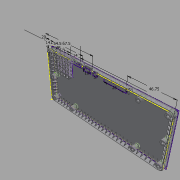
# Autodesk Inventor part: base
Saved by Autodesk Inventor 2019 (Build 230136000, 136)
## iProperties
Created: 2019-09-09
Part Number: base
Material: Generic
Document SubType Name: Modeling
Designer: jon
Density: 1 g/cm^3
Appearance: Default
Author: jon
Autodesk Inventor part; units mm, degrees
ref_plane "YZ Plane" through (0, 0, 0) normal (1, 0, 0) x (0, 1, 0)
ref_plane "XZ Plane" through (0, 0, 0) normal (0, 1, 0) x (-1, 0, 0)
ref_plane "XY Plane" through (0, 0, 0) normal (0, 0, 1) x (1, 0, 0)
sketch "Sketch1" plane through (0, 0, 0) normal (0, 0, 1) x (1, 0, 0)
  line L0 (0, 0) -> (154, 0)
  line L1 (154, 0) -> (154, 68)
  line L2 (154, 68) -> (0, 68)
  line L3 (0, 68) -> (0, 0)
  line L4 (1, 67) -> (153, 67)
  line L5 (153, 67) -> (153, 1)
  line L6 (153, 1) -> (1, 1)
  line L7 (1, 1) -> (1, 67)
  line L8 (1, 67) -> (8, 67)
  line L9 (1, 60) -> (1, 67)
  line L10 (1, 1) -> (8, 1)
  line L11 (1, 8) -> (1, 1)
  line L12 (153, 1) -> (146, 1)
  line L13 (153, 8) -> (153, 1)
  line L14 (153, 67) -> (146, 67)
  line L15 (153, 60) -> (153, 67)
  line L16 (30.5, 1) -> (37.5, 1)
  line L17 (116.5, 1) -> (123.5, 1)
  line L18 (116.5, 67) -> (123.5, 67)
  line L19 (30.5, 67) -> (37.5, 67)
  line L20 (1, 30.5) -> (1, 37.5)
  line L21 (153, 30.5) -> (153, 37.5)
  dimension "d0" = 154
  dimension "d1" = 68
  dimension "d2" = 1
  dimension "d3" = 1
  dimension "d4" = 1
  dimension "d123" = 1
  constraints: 44 end point, 10 horizontal, 6 point on line, 4 parallel, 2 perpendicular
  measures "d0" distance of L2.end L1.end
  measures "d1" distance of L1.end L0.end
  measures "d2" distance between parallel lines of L3 L7
  measures "d3" distance between parallel lines of L2 L4
  measures "d4" distance between parallel lines of L0 L6
  measures "d123" distance between parallel lines of L1 L5
extrude "Extrusion1" add sketch "Sketch1" along normal blind 6.4
extrude "Extrusion2" add sketch "Sketch1" against normal blind 1.3 contours L3 L2 L1 L0 | L4 L5 L6 L7
sketch "Sketch2" plane through (0, 0, 6.4) normal (0, 0, 1) x (1, 0, 0)
  line L0 (0, 68) -> (0, 0) projected
  line L1 (0, 0) -> (154, 0) projected
  line L2 (0, 68) -> (154, 68)
  line L3 (154, 68) -> (154, 0)
  line L4 (154, 0) -> (0, 0)
  line L5 (0, 0) -> (0, 68)
  line L6 (153.65, 67.65) -> (0.35, 67.65)
  line L7 (0.35, 67.65) -> (0.35, 0.35)
  line L8 (0.35, 0.35) -> (153.65, 0.35)
  line L9 (153.65, 0.35) -> (153.65, 67.65)
  dimension "d42" = 0.35
  constraints: 16 end point, 4 parallel, 2 perpendicular, 1 horizontal, 3 other
  measures "d42" distance between parallel lines of L2 L6
extrude "Extrusion3" cut sketch "Sketch2" against normal blind 1
fillet "Fillet2" radius 0.5 4 edges at (153, 34, 0) (77, 67, 0) (1, 34, 0) (77, 1, 0)
fillet "Fillet3" radius 4 8 edges at (152.8536, 1.1464, 0.1464) (153, 1, 3.45) (152.8536, 66.8536, 0.1464) (153, 67, 3.45) (1.1464, 1.1464, 0.1464) (1, 1, 3.45) (1.1464, 66.8536, 0.1464) (1, 67, 3.45)
fillet "Fillet9" radius 4.65 4 edges at (153.65, 0.35, 5.9) (153.65, 67.65, 5.9) (0.35, 67.65, 5.9) (0.35, 0.35, 5.9)
fillet "Fillet4" radius 5 4 edges at (154, 68, 2.05) (154, 0, 2.05) (0, 0, 2.05) (0, 68, 2.05)
sketch "Sketch10" plane through (0, 0, 0) normal (0, 0, 1) x (1, 0, 0)
  line L0 (149, 67) -> (5, 67) projected
  line L1 (5.25, 67) -> (4.75, 67)
  line L2 (4.75, 67) -> (4.75, 62)
  line L3 (4.75, 62) -> (5.25, 62)
  line L4 (5.25, 62) -> (5.25, 67)
  line L5 (0, 5) -> (0, 63) projected
  line L6 (5, 1) -> (149, 1) projected
  line L7 (5.25, 1) -> (4.75, 1)
  line L8 (4.75, 1) -> (4.75, 6)
  line L9 (4.75, 6) -> (5.25, 6)
  line L10 (5.25, 6) -> (5.25, 1)
  line L11 (10.215, 67) -> (9.715, 67)
  line L12 (9.715, 67) -> (9.715, 62)
  line L13 (9.715, 62) -> (10.215, 62)
  line L14 (10.215, 62) -> (10.215, 67)
  line L15 (10.215, 1) -> (9.715, 1)
  line L16 (9.715, 1) -> (9.715, 6)
  line L17 (9.715, 6) -> (10.215, 6)
  line L18 (10.215, 6) -> (10.215, 1)
  line L19 (15.18, 67) -> (14.68, 67)
  line L20 (14.68, 67) -> (14.68, 62)
  line L21 (14.68, 62) -> (15.18, 62)
  line L22 (15.18, 62) -> (15.18, 67)
  line L23 (15.18, 1) -> (14.68, 1)
  line L24 (14.68, 1) -> (14.68, 6)
  line L25 (14.68, 6) -> (15.18, 6)
  line L26 (15.18, 6) -> (15.18, 1)
  line L27 (20.145, 67) -> (19.645, 67)
  line L28 (19.645, 67) -> (19.645, 62)
  line L29 (19.645, 62) -> (20.145, 62)
  line L30 (20.145, 62) -> (20.145, 67)
  line L31 (20.145, 1) -> (19.645, 1)
  line L32 (19.645, 1) -> (19.645, 6)
  line L33 (19.645, 6) -> (20.145, 6)
  line L34 (20.145, 6) -> (20.145, 1)
  line L35 (25.11, 67) -> (24.61, 67)
  line L36 (24.61, 67) -> (24.61, 62)
  line L37 (24.61, 62) -> (25.11, 62)
  line L38 (25.11, 62) -> (25.11, 67)
  line L39 (25.11, 1) -> (24.61, 1)
  line L40 (24.61, 1) -> (24.61, 6)
  line L41 (24.61, 6) -> (25.11, 6)
  line L42 (25.11, 6) -> (25.11, 1)
  line L43 (30.075, 67) -> (29.575, 67)
  line L44 (29.575, 67) -> (29.575, 62)
  line L45 (29.575, 62) -> (30.075, 62)
  line L46 (30.075, 62) -> (30.075, 67)
  line L47 (30.075, 1) -> (29.575, 1)
  line L48 (29.575, 1) -> (29.575, 6)
  line L49 (29.575, 6) -> (30.075, 6)
  line L50 (30.075, 6) -> (30.075, 1)
  line L51 (35.04, 67) -> (34.54, 67)
  line L52 (34.54, 67) -> (34.54, 62)
  line L53 (34.54, 62) -> (35.04, 62)
  line L54 (35.04, 62) -> (35.04, 67)
  line L55 (35.04, 1) -> (34.54, 1)
  line L56 (34.54, 1) -> (34.54, 6)
  line L57 (34.54, 6) -> (35.04, 6)
  line L58 (35.04, 6) -> (35.04, 1)
  line L59 (40.005, 67) -> (39.505, 67)
  line L60 (39.505, 67) -> (39.505, 62)
  line L61 (39.505, 62) -> (40.005, 62)
  line L62 (40.005, 62) -> (40.005, 67)
  line L63 (40.005, 1) -> (39.505, 1)
  line L64 (39.505, 1) -> (39.505, 6)
  line L65 (39.505, 6) -> (40.005, 6)
  line L66 (40.005, 6) -> (40.005, 1)
  line L67 (44.97, 67) -> (44.47, 67)
  line L68 (44.47, 67) -> (44.47, 62)
  line L69 (44.47, 62) -> (44.97, 62)
  line L70 (44.97, 62) -> (44.97, 67)
  line L71 (44.97, 1) -> (44.47, 1)
  line L72 (44.47, 1) -> (44.47, 6)
  line L73 (44.47, 6) -> (44.97, 6)
  line L74 (44.97, 6) -> (44.97, 1)
  line L75 (49.935, 67) -> (49.435, 67)
  line L76 (49.435, 67) -> (49.435, 62)
  line L77 (49.435, 62) -> (49.935, 62)
  line L78 (49.935, 62) -> (49.935, 67)
  line L79 (49.935, 1) -> (49.435, 1)
  line L80 (49.435, 1) -> (49.435, 6)
  line L81 (49.435, 6) -> (49.935, 6)
  line L82 (49.935, 6) -> (49.935, 1)
  line L83 (54.9, 67) -> (54.4, 67)
  line L84 (54.4, 67) -> (54.4, 62)
  line L85 (54.4, 62) -> (54.9, 62)
  line L86 (54.9, 62) -> (54.9, 67)
  line L87 (54.9, 1) -> (54.4, 1)
  line L88 (54.4, 1) -> (54.4, 6)
  line L89 (54.4, 6) -> (54.9, 6)
  line L90 (54.9, 6) -> (54.9, 1)
  line L91 (59.865, 67) -> (59.365, 67)
  line L92 (59.365, 67) -> (59.365, 62)
  line L93 (59.365, 62) -> (59.865, 62)
  line L94 (59.865, 62) -> (59.865, 67)
  line L95 (59.865, 1) -> (59.365, 1)
  line L96 (59.365, 1) -> (59.365, 6)
  line L97 (59.365, 6) -> (59.865, 6)
  line L98 (59.865, 6) -> (59.865, 1)
  line L99 (64.83, 67) -> (64.33, 67)
  line L100 (64.33, 67) -> (64.33, 62)
  line L101 (64.33, 62) -> (64.83, 62)
  line L102 (64.83, 62) -> (64.83, 67)
  line L103 (64.83, 1) -> (64.33, 1)
  line L104 (64.33, 1) -> (64.33, 6)
  line L105 (64.33, 6) -> (64.83, 6)
  line L106 (64.83, 6) -> (64.83, 1)
  line L107 (69.795, 67) -> (69.295, 67)
  line L108 (69.295, 67) -> (69.295, 62)
  line L109 (69.295, 62) -> (69.795, 62)
  line L110 (69.795, 62) -> (69.795, 67)
  line L111 (69.795, 1) -> (69.295, 1)
  line L112 (69.295, 1) -> (69.295, 6)
  line L113 (69.295, 6) -> (69.795, 6)
  line L114 (69.795, 6) -> (69.795, 1)
  line L115 (74.76, 67) -> (74.26, 67)
  line L116 (74.26, 67) -> (74.26, 62)
  line L117 (74.26, 62) -> (74.76, 62)
  line L118 (74.76, 62) -> (74.76, 67)
  line L119 (74.76, 1) -> (74.26, 1)
  line L120 (74.26, 1) -> (74.26, 6)
  line L121 (74.26, 6) -> (74.76, 6)
  line L122 (74.76, 6) -> (74.76, 1)
  line L123 (79.725, 67) -> (79.225, 67)
  line L124 (79.225, 67) -> (79.225, 62)
  line L125 (79.225, 62) -> (79.725, 62)
  line L126 (79.725, 62) -> (79.725, 67)
  line L127 (79.725, 1) -> (79.225, 1)
  line L128 (79.225, 1) -> (79.225, 6)
  line L129 (79.225, 6) -> (79.725, 6)
  line L130 (79.725, 6) -> (79.725, 1)
  line L131 (84.69, 67) -> (84.19, 67)
  line L132 (84.19, 67) -> (84.19, 62)
  line L133 (84.19, 62) -> (84.69, 62)
  line L134 (84.69, 62) -> (84.69, 67)
  line L135 (84.69, 1) -> (84.19, 1)
  line L136 (84.19, 1) -> (84.19, 6)
  line L137 (84.19, 6) -> (84.69, 6)
  line L138 (84.69, 6) -> (84.69, 1)
  line L139 (89.655, 67) -> (89.155, 67)
  line L140 (89.155, 67) -> (89.155, 62)
  line L141 (89.155, 62) -> (89.655, 62)
  line L142 (89.655, 62) -> (89.655, 67)
  line L143 (89.655, 1) -> (89.155, 1)
  line L144 (89.155, 1) -> (89.155, 6)
  line L145 (89.155, 6) -> (89.655, 6)
  line L146 (89.655, 6) -> (89.655, 1)
  line L147 (94.62, 67) -> (94.12, 67)
  line L148 (94.12, 67) -> (94.12, 62)
  line L149 (94.12, 62) -> (94.62, 62)
  line L150 (94.62, 62) -> (94.62, 67)
  line L151 (94.62, 1) -> (94.12, 1)
  line L152 (94.12, 1) -> (94.12, 6)
  line L153 (94.12, 6) -> (94.62, 6)
  line L154 (94.62, 6) -> (94.62, 1)
  line L155 (99.585, 67) -> (99.085, 67)
  line L156 (99.085, 67) -> (99.085, 62)
  line L157 (99.085, 62) -> (99.585, 62)
  line L158 (99.585, 62) -> (99.585, 67)
  line L159 (99.585, 1) -> (99.085, 1)
  line L160 (99.085, 1) -> (99.085, 6)
  line L161 (99.085, 6) -> (99.585, 6)
  line L162 (99.585, 6) -> (99.585, 1)
  line L163 (104.55, 67) -> (104.05, 67)
  line L164 (104.05, 67) -> (104.05, 62)
  line L165 (104.05, 62) -> (104.55, 62)
  line L166 (104.55, 62) -> (104.55, 67)
  line L167 (104.55, 1) -> (104.05, 1)
  line L168 (104.05, 1) -> (104.05, 6)
  line L169 (104.05, 6) -> (104.55, 6)
  line L170 (104.55, 6) -> (104.55, 1)
  line L171 (109.515, 67) -> (109.015, 67)
  line L172 (109.015, 67) -> (109.015, 62)
  line L173 (109.015, 62) -> (109.515, 62)
  line L174 (109.515, 62) -> (109.515, 67)
  line L175 (109.515, 1) -> (109.015, 1)
  line L176 (109.015, 1) -> (109.015, 6)
  line L177 (109.015, 6) -> (109.515, 6)
  line L178 (109.515, 6) -> (109.515, 1)
  line L179 (114.48, 67) -> (113.98, 67)
  line L180 (113.98, 67) -> (113.98, 62)
  line L181 (113.98, 62) -> (114.48, 62)
  line L182 (114.48, 62) -> (114.48, 67)
  line L183 (114.48, 1) -> (113.98, 1)
  line L184 (113.98, 1) -> (113.98, 6)
  line L185 (113.98, 6) -> (114.48, 6)
  line L186 (114.48, 6) -> (114.48, 1)
  line L187 (119.445, 67) -> (118.945, 67)
  line L188 (118.945, 67) -> (118.945, 62)
  line L189 (118.945, 62) -> (119.445, 62)
  line L190 (119.445, 62) -> (119.445, 67)
  line L191 (119.445, 1) -> (118.945, 1)
  line L192 (118.945, 1) -> (118.945, 6)
  line L193 (118.945, 6) -> (119.445, 6)
  line L194 (119.445, 6) -> (119.445, 1)
  line L195 (124.41, 67) -> (123.91, 67)
  line L196 (123.91, 67) -> (123.91, 62)
  line L197 (123.91, 62) -> (124.41, 62)
  line L198 (124.41, 62) -> (124.41, 67)
  line L199 (124.41, 1) -> (123.91, 1)
  line L200 (123.91, 1) -> (123.91, 6)
  line L201 (123.91, 6) -> (124.41, 6)
  line L202 (124.41, 6) -> (124.41, 1)
  line L203 (129.375, 67) -> (128.875, 67)
  line L204 (128.875, 67) -> (128.875, 62)
  line L205 (128.875, 62) -> (129.375, 62)
  line L206 (129.375, 62) -> (129.375, 67)
  line L207 (129.375, 1) -> (128.875, 1)
  line L208 (128.875, 1) -> (128.875, 6)
  line L209 (128.875, 6) -> (129.375, 6)
  line L210 (129.375, 6) -> (129.375, 1)
  line L211 (134.34, 67) -> (133.84, 67)
  line L212 (133.84, 67) -> (133.84, 62)
  line L213 (133.84, 62) -> (134.34, 62)
  line L214 (134.34, 62) -> (134.34, 67)
  line L215 (134.34, 1) -> (133.84, 1)
  line L216 (133.84, 1) -> (133.84, 6)
  line L217 (133.84, 6) -> (134.34, 6)
  line L218 (134.34, 6) -> (134.34, 1)
  line L219 (139.305, 67) -> (138.805, 67)
  line L220 (138.805, 67) -> (138.805, 62)
  line L221 (138.805, 62) -> (139.305, 62)
  line L222 (139.305, 62) -> (139.305, 67)
  line L223 (139.305, 1) -> (138.805, 1)
  line L224 (138.805, 1) -> (138.805, 6)
  line L225 (138.805, 6) -> (139.305, 6)
  line L226 (139.305, 6) -> (139.305, 1)
  line L227 (144.27, 67) -> (143.77, 67)
  line L228 (143.77, 67) -> (143.77, 62)
  line L229 (143.77, 62) -> (144.27, 62)
  line L230 (144.27, 62) -> (144.27, 67)
  line L231 (144.27, 1) -> (143.77, 1)
  line L232 (143.77, 1) -> (143.77, 6)
  line L233 (143.77, 6) -> (144.27, 6)
  line L234 (144.27, 6) -> (144.27, 1)
  line L235 (149.235, 67) -> (148.735, 67)
  line L236 (148.735, 67) -> (148.735, 62)
  line L237 (148.735, 62) -> (149.235, 62)
  line L238 (149.235, 62) -> (149.235, 67)
  line L239 (149.235, 1) -> (148.735, 1)
  line L240 (148.735, 1) -> (148.735, 6)
  line L241 (148.735, 6) -> (149.235, 6)
  line L242 (149.235, 6) -> (149.235, 1)
  point P0 (0, 0)
  dimension "d144" = 0.5
  dimension "d145" = 5
  dimension "d146" = 4.75
  dimension "d147" = 0.5
  dimension "d148" = 5
  dimension "d151" = 4.965
  constraints: 480 end point, 4 parallel, 3 horizontal, 2 perpendicular, 2 point on line, 464 other
  measures "d144" distance of L3.end L2.end
  measures "d145" distance of L2.end L1.end
  measures "d146" distance between parallel lines of L2 L5
  measures "d147" distance of L8.end L9.end
  measures "d148" distance of L7.end L8.end
  measures "d151" distance of L1.start L11.start
extrude "Extrusion10" add sketch "Sketch10" along normal blind 5
sketch "Sketch11" plane through (0, 0, 0) normal (0, 0, 1) x (1, 0, 0)
  line L0 (1, 5) -> (1, 63) projected
  line L1 (1, 5.25) -> (6, 5.25)
  line L2 (6, 5.25) -> (6, 4.75)
  line L3 (6, 4.75) -> (1, 4.75)
  line L4 (1, 4.75) -> (1, 5.25)
  line L5 (149, 0) -> (5, 0) projected
  line L6 (153, 5) -> (153, 63) projected
  line L7 (153, 5.25) -> (148, 5.25)
  line L8 (148, 5.25) -> (148, 4.75)
  line L9 (148, 4.75) -> (153, 4.75)
  line L10 (153, 4.75) -> (153, 5.25)
  line L11 (1, 10.085) -> (6, 10.085)
  line L12 (6, 10.085) -> (6, 9.585)
  line L13 (6, 9.585) -> (1, 9.585)
  line L14 (1, 9.585) -> (1, 10.085)
  line L15 (153, 10.085) -> (148, 10.085)
  line L16 (148, 10.085) -> (148, 9.585)
  line L17 (148, 9.585) -> (153, 9.585)
  line L18 (153, 9.585) -> (153, 10.085)
  line L19 (1, 14.92) -> (6, 14.92)
  line L20 (6, 14.92) -> (6, 14.42)
  line L21 (6, 14.42) -> (1, 14.42)
  line L22 (1, 14.42) -> (1, 14.92)
  line L23 (153, 14.92) -> (148, 14.92)
  line L24 (148, 14.92) -> (148, 14.42)
  line L25 (148, 14.42) -> (153, 14.42)
  line L26 (153, 14.42) -> (153, 14.92)
  line L27 (1, 19.755) -> (6, 19.755)
  line L28 (6, 19.755) -> (6, 19.255)
  line L29 (6, 19.255) -> (1, 19.255)
  line L30 (1, 19.255) -> (1, 19.755)
  line L31 (153, 19.755) -> (148, 19.755)
  line L32 (148, 19.755) -> (148, 19.255)
  line L33 (148, 19.255) -> (153, 19.255)
  line L34 (153, 19.255) -> (153, 19.755)
  line L35 (1, 24.59) -> (6, 24.59)
  line L36 (6, 24.59) -> (6, 24.09)
  line L37 (6, 24.09) -> (1, 24.09)
  line L38 (1, 24.09) -> (1, 24.59)
  line L39 (153, 24.59) -> (148, 24.59)
  line L40 (148, 24.59) -> (148, 24.09)
  line L41 (148, 24.09) -> (153, 24.09)
  line L42 (153, 24.09) -> (153, 24.59)
  line L43 (1, 29.425) -> (6, 29.425)
  line L44 (6, 29.425) -> (6, 28.925)
  line L45 (6, 28.925) -> (1, 28.925)
  line L46 (1, 28.925) -> (1, 29.425)
  line L47 (153, 29.425) -> (148, 29.425)
  line L48 (148, 29.425) -> (148, 28.925)
  line L49 (148, 28.925) -> (153, 28.925)
  line L50 (153, 28.925) -> (153, 29.425)
  line L51 (1, 34.26) -> (6, 34.26)
  line L52 (6, 34.26) -> (6, 33.76)
  line L53 (6, 33.76) -> (1, 33.76)
  line L54 (1, 33.76) -> (1, 34.26)
  line L55 (153, 34.26) -> (148, 34.26)
  line L56 (148, 34.26) -> (148, 33.76)
  line L57 (148, 33.76) -> (153, 33.76)
  line L58 (153, 33.76) -> (153, 34.26)
  line L59 (1, 39.095) -> (6, 39.095)
  line L60 (6, 39.095) -> (6, 38.595)
  line L61 (6, 38.595) -> (1, 38.595)
  line L62 (1, 38.595) -> (1, 39.095)
  line L63 (153, 39.095) -> (148, 39.095)
  line L64 (148, 39.095) -> (148, 38.595)
  line L65 (148, 38.595) -> (153, 38.595)
  line L66 (153, 38.595) -> (153, 39.095)
  line L67 (1, 43.93) -> (6, 43.93)
  line L68 (6, 43.93) -> (6, 43.43)
  line L69 (6, 43.43) -> (1, 43.43)
  line L70 (1, 43.43) -> (1, 43.93)
  line L71 (153, 43.93) -> (148, 43.93)
  line L72 (148, 43.93) -> (148, 43.43)
  line L73 (148, 43.43) -> (153, 43.43)
  line L74 (153, 43.43) -> (153, 43.93)
  line L75 (1, 48.765) -> (6, 48.765)
  line L76 (6, 48.765) -> (6, 48.265)
  line L77 (6, 48.265) -> (1, 48.265)
  line L78 (1, 48.265) -> (1, 48.765)
  line L79 (153, 48.765) -> (148, 48.765)
  line L80 (148, 48.765) -> (148, 48.265)
  line L81 (148, 48.265) -> (153, 48.265)
  line L82 (153, 48.265) -> (153, 48.765)
  line L83 (1, 53.6) -> (6, 53.6)
  line L84 (6, 53.6) -> (6, 53.1)
  line L85 (6, 53.1) -> (1, 53.1)
  line L86 (1, 53.1) -> (1, 53.6)
  line L87 (153, 53.6) -> (148, 53.6)
  line L88 (148, 53.6) -> (148, 53.1)
  line L89 (148, 53.1) -> (153, 53.1)
  line L90 (153, 53.1) -> (153, 53.6)
  line L91 (1, 58.435) -> (6, 58.435)
  line L92 (6, 58.435) -> (6, 57.935)
  line L93 (6, 57.935) -> (1, 57.935)
  line L94 (1, 57.935) -> (1, 58.435)
  line L95 (153, 58.435) -> (148, 58.435)
  line L96 (148, 58.435) -> (148, 57.935)
  line L97 (148, 57.935) -> (153, 57.935)
  line L98 (153, 57.935) -> (153, 58.435)
  line L99 (1, 63.27) -> (6, 63.27)
  line L100 (6, 63.27) -> (6, 62.77)
  line L101 (6, 62.77) -> (1, 62.77)
  line L102 (1, 62.77) -> (1, 63.27)
  line L103 (153, 63.27) -> (148, 63.27)
  line L104 (148, 63.27) -> (148, 62.77)
  line L105 (148, 62.77) -> (153, 62.77)
  line L106 (153, 62.77) -> (153, 63.27)
  point P0 (0, 0)
  dimension "d161" = 5
  dimension "d162" = 0.5
  dimension "d163" = 4.75
  dimension "d164" = 5
  dimension "d165" = 0.5
  dimension "d168" = 4.835
  constraints: 208 end point, 4 parallel, 2 horizontal, 2 perpendicular, 2 point on line, 1 vertical, 192 other
  measures "d161" distance of L2.end L3.end
  measures "d162" distance of L1.end L2.end
  measures "d163" distance between parallel lines of L5 L3
  measures "d164" distance of L9.end L8.end
  measures "d165" distance of L8.end L7.end
  measures "d168" distance of L1.start L11.start
extrude "Extrusion11" add sketch "Sketch11" along normal blind 5
fillet "Fillet5" radius 1.75 8 edges at (152.5355, 66.5355, -1.3) (154, 34, -1.3) (152.5355, 1.4645, -1.3) (77, 0, -1.3) (1.4645, 1.4645, -1.3) (0, 34, -1.3) (1.4645, 66.5355, -1.3) (77, 68, -1.3)
sketch "Sketch4" plane through (0, 0, -1.3) normal (0, 0, -1) x (-1, 0, 0)
  line L0 (0, 0) -> (0, 68) projected
  line L1 (-154, 0) -> (0, 0) projected
  circle A0 centre (-149, 5) radius 2.75
  circle A1 centre (-120, 5) radius 2.75
  circle A2 centre (-34, 5) radius 2.75
  circle A3 centre (-5, 5) radius 2.75
  circle A4 centre (-5, 63) radius 2.75
  circle A5 centre (-34, 63) radius 2.75
  circle A6 centre (-120, 63) radius 2.75
  circle A7 centre (-149, 63) radius 2.75
  circle A8 centre (-149, 34) radius 2.75
  circle A9 centre (-5, 34) radius 2.75
  dimension "d43" = 29
  dimension "d44" = 86
  dimension "d45" = 29
  dimension "d46" = 29
  dimension "d47" = 29
  dimension "d48" = 29
  dimension "d49" = 86
  dimension "d50" = 29
  dimension "d51" = 29
  dimension "d52" = 5
  dimension "d53" = 5
  dimension "d124" = 5.5
  dimension "d125" = 5.5
  dimension "d126" = 5.5
  dimension "d127" = 5.5
  dimension "d128" = 5.5
  dimension "d129" = 5.5
  dimension "d130" = 5.5
  dimension "d131" = 5.5
  dimension "d132" = 5.5
  dimension "d133" = 5.5
  constraints: 10 centre point, 10 coincident
  measures "d43" distance of point (-5, 5) point (-34, 5)
  measures "d44" distance of point (-34, 5) point (-120, 5)
  measures "d45" distance of point (-149, 5) point (-120, 5)
  measures "d46" distance of point (-149, 34) point (-149, 5)
  measures "d47" distance of point (-149, 63) point (-149, 34)
  measures "d48" distance of point (-120, 63) point (-149, 63)
  measures "d49" distance of point (-34, 63) point (-120, 63)
  measures "d50" distance of point (-5, 34) point (-5, 5)
  measures "d51" distance of point (-5, 34) point (-5, 63)
  measures "d52" distance from line of L0 point (-5, 5)
  measures "d53" distance from line of L1 point (-5, 5)
  measures "d124" diameter of A0
  measures "d125" diameter of A1
  measures "d126" diameter of A2
  measures "d127" diameter of A3
  measures "d128" diameter of A4
  measures "d129" diameter of A5
  measures "d130" diameter of A6
  measures "d131" diameter of A7
  measures "d132" diameter of A8
  measures "d133" diameter of A9
extrude "Extrusion8" add sketch "Sketch4" against normal blind 7.75
hole "Hole1" at (149, 63, -1.3) at (120, 63, -1.3) at (34, 63, -1.3) at (5, 63, -1.3) at (5, 34, -1.3) at (5, 5, -1.3) at (34, 5, -1.3) at (120, 5, -1.3) at (149, 5, -1.3) at (149, 34, -1.3) direction (0, 0, 1) diameter 2.9 end through all counterbore diameter 5 counterbore depth 3 clearance for "Hex Head Machine Screw" size "M2.5" standard "Ansi Metric M Profile"
fillet "Fillet6" radius 0.25 10 edges at (149, 60.5, -1.3) (149, 31.5, -1.3) (149, 2.5, -1.3) (120, 2.5, -1.3) (120, 60.5, -1.3) (34, 60.5, -1.3) (34, 2.5, -1.3) (5, 2.5, -1.3) (5, 31.5, -1.3) (5, 60.5, -1.3)
chamfer "Chamfer2" distance 4 angle 45 52 edges at (9.965, 62, 5) (14.93, 62, 5) (19.895, 62, 5) (24.86, 62, 5) (29.825, 62, 5) (39.755, 62, 5) (44.72, 62, 5) (49.685, 62, 5) (54.65, 62, 5) (59.615, 62, 5) (64.58, 62, 5) (69.545, 62, 5) (74.51, 62, 5) (79.475, 62, 5) (84.44, 62, 5) (89.405, 62, 5) (94.37, 62, 5) (99.335, 62, 5) (104.3, 62, 5) (109.265, 62, 5) (114.23, 62, 5) (124.16, 62, 5) (129.125, 62, 5) (134.09, 62, 5) (139.055, 62, 5) (144.02, 62, 5) (9.965, 6, 5) (14.93, 6, 5) (19.895, 6, 5) (24.86, 6, 5) (29.825, 6, 5) (39.755, 6, 5) (44.72, 6, 5) (49.685, 6, 5) (54.65, 6, 5) (59.615, 6, 5) (64.58, 6, 5) (69.545, 6, 5) (74.51, 6, 5) (79.475, 6, 5) (84.44, 6, 5) (89.405, 6, 5) (94.37, 6, 5) (99.335, 6, 5) (104.3, 6, 5) (109.265, 6, 5) (114.23, 6, 5) (124.16, 6, 5) (129.125, 6, 5) (134.09, 6, 5) (139.055, 6, 5) (144.02, 6, 5)
chamfer "Chamfer3" distance 4 angle 45 20 edges at (6, 9.835, 5) (6, 14.67, 5) (6, 19.505, 5) (6, 24.34, 5) (6, 29.175, 5) (6, 38.845, 5) (6, 43.68, 5) (6, 48.515, 5) (6, 53.35, 5) (6, 58.185, 5) (148, 58.185, 5) (148, 53.35, 5) (148, 48.515, 5) (148, 43.68, 5) (148, 38.845, 5) (148, 29.175, 5) (148, 24.34, 5) (148, 19.505, 5) (148, 14.67, 5) (148, 9.835, 5)
sketch "Sketch12" plane through (0, 0, 6.4) normal (0, 0, 1) x (1, 0, 0)
  line L0 (5, 68) -> (149, 68) projected
  line L1 (37, 68) -> (51, 68)
  line L2 (51, 68) -> (51, 64.5)
  line L3 (51, 64.5) -> (37, 64.5)
  line L4 (37, 64.5) -> (37, 68)
  line L5 (0, 5) -> (0, 63) projected
  line L6 (5, 68) -> (149, 68) projected
  line L7 (54.5, 68) -> (64.5, 68)
  line L8 (64.5, 68) -> (64.5, 63.9)
  line L9 (64.5, 63.9) -> (54.5, 63.9)
  line L10 (54.5, 63.9) -> (54.5, 68)
  line L11 (67.5, 68) -> (72.5, 68)
  line L12 (72.5, 68) -> (72.5, 64)
  line L13 (72.5, 64) -> (67.5, 64)
  line L14 (67.5, 64) -> (67.5, 68)
  line L15 (81.25, 67.75) -> (107.25, 67.75)
  line L16 (107.25, 67.75) -> (107.25, 63.75)
  line L17 (107.25, 63.75) -> (81.25, 63.75)
  line L18 (81.25, 63.75) -> (81.25, 67.75)
  line L19 (154, 63) -> (154, 5) projected
  point P0 (0, 0)
  dimension "d178" = 37
  dimension "d179" = 14
  dimension "d182" = 10
  dimension "d183" = 4.1
  dimension "d184" = 3.5
  dimension "d185" = 54.5
  dimension "d186" = 5
  dimension "d187" = 4
  dimension "d188" = 67.5
  dimension "d195" = 26
  dimension "d196" = 4
  dimension "d197" = 46.75
  dimension "d200" = 0.25
  constraints: 32 end point, 8 parallel, 4 horizontal, 4 perpendicular, 3 point on line
  measures "d178" distance between parallel lines of L5 L4
  measures "d179" distance between parallel lines of L2 L4
  measures "d182" distance of L8.end L9.end
  measures "d183" distance of L7.end L8.end
  measures "d184" distance between parallel lines of L0 L3
  measures "d185" distance between parallel lines of L5 L10
  measures "d186" distance of L12.end L13.end
  measures "d187" distance of L11.end L12.end
  measures "d188" distance between parallel lines of L5 L14
  measures "d195" distance of L16.end L17.end
  measures "d196" distance of L15.end L16.end
  measures "d197" distance between parallel lines of L19 L16
  measures "d200" distance between parallel lines of L6 L15
extrude "Extrusion12" cut sketch "Sketch12" against normal blind 2 contours L0 L12 L13 L14
extrude "Extrusion13" cut sketch "Sketch12" against normal blind 3.5 contours L0 L8 L9 L10
fillet "Fillet10" radius 0.75 2 edges at (64.5, 65.95, 2.9) (54.5, 65.95, 2.9)
sketch "Sketch14" plane through (0, 0, 0) normal (0, 0, 1) x (1, 0, 0)
  line L0 (8.35, 65.65) -> (9.15, 65.65)
  line L1 (9.15, 65.65) -> (9.15, 42.35)
  line L2 (9.15, 42.35) -> (8.35, 42.35)
  line L3 (8.35, 42.35) -> (8.35, 65.65)
  line L4 (12.85, 65.65) -> (13.65, 65.65)
  line L5 (13.65, 65.65) -> (13.65, 42.35)
  line L6 (13.65, 42.35) -> (12.85, 42.35)
  line L7 (12.85, 42.35) -> (12.85, 65.65)
  line L8 (17.35, 65.65) -> (18.15, 65.65)
  line L9 (18.15, 65.65) -> (18.15, 42.35)
  line L10 (18.15, 42.35) -> (17.35, 42.35)
  line L11 (17.35, 42.35) -> (17.35, 65.65)
  line L12 (21.85, 65.65) -> (22.65, 65.65)
  line L13 (22.65, 65.65) -> (22.65, 42.35)
  line L14 (22.65, 42.35) -> (21.85, 42.35)
  line L15 (21.85, 42.35) -> (21.85, 65.65)
  line L16 (26.35, 65.65) -> (27.15, 65.65)
  line L17 (27.15, 65.65) -> (27.15, 42.35)
  line L18 (27.15, 42.35) -> (26.35, 42.35)
  line L19 (26.35, 42.35) -> (26.35, 65.65)
  line L20 (30.85, 65.65) -> (31.65, 65.65)
  line L21 (31.65, 65.65) -> (31.65, 42.35)
  line L22 (31.65, 42.35) -> (30.85, 42.35)
  line L23 (30.85, 42.35) -> (30.85, 65.65)
  line L24 (8.35, 65.65) -> (31.65, 65.65)
  line L25 (31.65, 65.65) -> (31.65, 64.85)
  line L26 (31.65, 64.85) -> (8.35, 64.85)
  line L27 (8.35, 64.85) -> (8.35, 65.65)
  line L28 (31.65, 61.15) -> (31.65, 60.35)
  line L29 (30.85, 61.15) -> (31.65, 61.15)
  line L30 (26.35, 61.15) -> (27.15, 61.15)
  line L31 (21.85, 61.15) -> (22.65, 61.15)
  line L32 (17.35, 61.15) -> (18.15, 61.15)
  line L33 (12.85, 61.15) -> (13.65, 61.15)
  line L34 (31.65, 60.35) -> (8.35, 60.35)
  line L35 (8.35, 61.15) -> (31.65, 61.15)
  line L36 (8.35, 60.35) -> (8.35, 61.15)
  line L37 (8.35, 61.15) -> (9.15, 61.15)
  line L38 (31.65, 56.65) -> (31.65, 55.85)
  line L39 (30.85, 56.65) -> (31.65, 56.65)
  line L40 (26.35, 56.65) -> (27.15, 56.65)
  line L41 (21.85, 56.65) -> (22.65, 56.65)
  line L42 (17.35, 56.65) -> (18.15, 56.65)
  line L43 (12.85, 56.65) -> (13.65, 56.65)
  line L44 (31.65, 55.85) -> (8.35, 55.85)
  line L45 (8.35, 56.65) -> (31.65, 56.65)
  line L46 (8.35, 55.85) -> (8.35, 56.65)
  line L47 (8.35, 56.65) -> (9.15, 56.65)
  line L48 (31.65, 52.15) -> (31.65, 51.35)
  line L49 (30.85, 52.15) -> (31.65, 52.15)
  line L50 (26.35, 52.15) -> (27.15, 52.15)
  line L51 (21.85, 52.15) -> (22.65, 52.15)
  line L52 (17.35, 52.15) -> (18.15, 52.15)
  line L53 (12.85, 52.15) -> (13.65, 52.15)
  line L54 (31.65, 51.35) -> (8.35, 51.35)
  line L55 (8.35, 52.15) -> (31.65, 52.15)
  line L56 (8.35, 51.35) -> (8.35, 52.15)
  line L57 (8.35, 52.15) -> (9.15, 52.15)
  line L58 (31.65, 47.65) -> (31.65, 46.85)
  line L59 (30.85, 47.65) -> (31.65, 47.65)
  line L60 (26.35, 47.65) -> (27.15, 47.65)
  line L61 (21.85, 47.65) -> (22.65, 47.65)
  line L62 (17.35, 47.65) -> (18.15, 47.65)
  line L63 (12.85, 47.65) -> (13.65, 47.65)
  line L64 (31.65, 46.85) -> (8.35, 46.85)
  line L65 (8.35, 47.65) -> (31.65, 47.65)
  line L66 (8.35, 46.85) -> (8.35, 47.65)
  line L67 (8.35, 47.65) -> (9.15, 47.65)
  line L68 (31.65, 43.15) -> (31.65, 42.35)
  line L69 (30.85, 43.15) -> (31.65, 43.15)
  line L70 (26.35, 43.15) -> (27.15, 43.15)
  line L71 (21.85, 43.15) -> (22.65, 43.15)
  line L72 (17.35, 43.15) -> (18.15, 43.15)
  line L73 (12.85, 43.15) -> (13.65, 43.15)
  line L74 (31.65, 42.35) -> (8.35, 42.35)
  line L75 (8.35, 43.15) -> (31.65, 43.15)
  line L76 (8.35, 42.35) -> (8.35, 43.15)
  line L77 (8.35, 43.15) -> (9.15, 43.15)
  line L78 (5, 68) -> (67.5, 68) projected
  line L79 (0, 5) -> (0, 63) projected
  point P0 (0, 0)
  point P1 (36, 68)
  point P2 (20, 54)
  dimension "d218" = 0.8
  dimension "d219" = 23.3
  dimension "d222" = 4.5
  dimension "d227" = 0.8
  dimension "d230" = 4.5
  dimension "d237" = 11.65
  dimension "d238" = 11.65
  dimension "d239" = 20
  dimension "d240" = 14
  constraints: 156 end point, 4 parallel, 3 horizontal, 2 collinear, 2 perpendicular, 1 point on line, 1 vertical, 163 other
  measures "d218" distance of L1.end L2.end
  measures "d219" distance of L0.end L1.end
  measures "d222" distance of L0.start L4.start
  measures "d227" distance of L24.end L25.end
  measures "d230" distance of L24.end L28.start
  measures "d237" distance from line of point (20, 54) L3
  measures "d238" distance from line of point (20, 54) L24
  measures "d239" distance from line of point (20, 54) L79
  measures "d240" distance from line of point (20, 54) L78
extrude "Extrusion15" add sketch "Sketch14" along normal blind 5.55 contours L0 L1 L26 L3 | L24 L7 L26 L1 | L26 L1 L35 L3 | L4 L5 L26 L7 | L35 L1 L34 L3 | L35 L7 L34 L1 | L26 L5 L33 L7 | L24 L11 L26 L5 | L34 L1 L45 L3 | L33 L5 L34 L7 | L8 L9 L26 L11 | L45 L1 L44 L3 | L45 L7 L44 L1 | L34 L5 L43 L7 | L35 L11 L34 L5 | L26 L9 L32 L11 | L24 L15 L26 L9 | L44 L1 L55 L3 | L43 L5 L44 L7 | L32 L9 L34 L11 | L12 L13 L26 L15 | L55 L1 L54 L3 | L55 L7 L54 L1 | L44 L5 L53 L7 | L45 L11 L44 L5 | L34 L9 L42 L11 | L35 L15 L34 L9 | L26 L13 L31 L15 | L24 L19 L26 L13 | L54 L1 L65 L3 | L53 L5 L54 L7 | L42 L9 L44 L11 | L31 L13 L34 L15 | L16 L17 L26 L19 | L65 L1 L64 L3 | L65 L7 L64 L1 | L54 L5 L63 L7 | L55 L11 L54 L5 | L44 L9 L52 L11 | L45 L15 L44 L9 | L34 L13 L41 L15 | L35 L19 L34 L13 | L26 L17 L30 L19 | L24 L23 L26 L17 | L64 L1 L75 L3 | L63 L5 L64 L7 | L52 L9 L54 L11 | L41 L13 L44 L15 | L30 L17 L34 L19 | L20 L21 L26 L23 | L75 L1 L2 L3 | L75 L7 L74 L1 | L64 L5 L73 L7 | L65 L11 L64 L5 | L54 L9 L62 L11 | L55 L15 L54 L9 | L44 L13 L51 L15 | L45 L19 L44 L13 | L34 L17 L40 L19 | L35 L23 L34 L17 | L26 L21 L29 L23 | L73 L5 L6 L7 | L62 L9 L64 L11 | L51 L13 L54 L15 | L40 L17 L44 L19 | L29 L21 L34 L23 | L75 L11 L74 L5 | L64 L9 L72 L11 | L65 L15 L64 L9 | L54 L13 L61 L15 | L55 L19 L54 L13 | L44 L17 L50 L19 | L45 L23 L44 L17 | L34 L21 L39 L23 | L72 L9 L10 L11 | L61 L13 L64 L15 | L50 L17 L54 L19 | L39 L21 L44 L23 | L75 L15 L74 L9 | L64 L13 L71 L15 | L65 L19 L64 L13 | L54 L17 L60 L19 | L55 L23 L54 L17 | L44 L21 L49 L23 | L71 L13 L14 L15 | L60 L17 L64 L19 | L49 L21 L54 L23 | L75 L19 L74 L13 | L64 L17 L70 L19 | L65 L23 L64 L17 | L54 L21 L59 L23 | L70 L17 L18 L19 | L59 L21 L64 L23 | L75 L23 L74 L17 | L64 L21 L69 L23 | L69 L21 L22 L23
sketch "Sketch16" plane through (0, 0, 5.55) normal (0, 0, 1) x (1, 0, 0)
  line L0 (15.5, 58.5) -> (24.5, 58.5)
  line L1 (24.5, 58.5) -> (24.5, 49.5)
  line L2 (24.5, 49.5) -> (15.5, 49.5)
  line L3 (15.5, 49.5) -> (15.5, 58.5)
  line L4 (31.65, 65.65) -> (8.35, 65.65) projected
  line L5 (8.35, 65.65) -> (8.35, 42.35) projected
  point P0 (0, 0)
  dimension "d249" = 9
  dimension "d250" = 9
  dimension "d251" = 7.15
  dimension "d252" = 7.15
  constraints: 8 end point, 2 parallel, 1 horizontal, 1 perpendicular
  measures "d249" distance of L1.end L2.end
  measures "d250" distance of L0.end L1.end
  measures "d251" distance between parallel lines of L4 L0
  measures "d252" distance between parallel lines of L5 L3
extrude "Extrusion17" cut sketch "Sketch16" against normal blind 0.5
chamfer "Chamfer5" distance 0.5 distance2 1 10 edges at (29.75, 67.65, 6.4) (66, 67.65, 6.4) (110.75, 67.65, 6.4) (152.288, 66.288, 6.4) (153.65, 34, 6.4) (152.288, 1.712, 6.4) (77, 0.35, 6.4) (1.712, 1.712, 6.4) (0.35, 34, 6.4) (1.712, 66.288, 6.4) measured on face at (1.7827, 66.2173, 6.4) measured on face at (151.9345, 2.0655, 6.4) measured on face at (66, 67.55, 6.4) measured on face at (153.55, 34, 6.4) measured on face at (77, 0.85, 6.4) measured on face at (152.2173, 66.2173, 6.4) measured on face at (110.75, 67.15, 6.4) measured on face at (0.85, 34, 6.4) measured on face at (2.0655, 2.0655, 6.4) measured on face at (29.75, 67.55, 6.4)
extrude "Extrusion18" cut sketch "Sketch12" against normal blind 2.75 contours L0 L2 L3 L4
body "Solid1"
